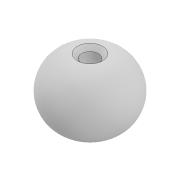
# Autodesk Inventor part: seventh
Saved by Autodesk Inventor 2020 (Build 240168000, 168)
## iProperties
Created: 2021-12-10
Part Number: seventh
Material: Generic
Document SubType Name: Modeling
Designer: NIKHIL VINOD
Density: 1 g/cm^3
Appearance: Default
Author: NIKHIL VINOD
Autodesk Inventor part; units mm, degrees
ref_plane "YZ Plane" through (0, 0, 0) normal (1, 0, 0) x (0, 1, 0)
ref_plane "XZ Plane" through (0, 0, 0) normal (0, 1, 0) x (-1, 0, 0)
ref_plane "XY Plane" through (0, 0, 0) normal (0, 0, 1) x (1, 0, 0)
sketch "Sketch1" plane through (0, 0, 0) normal (0, 0, 1) x (1, 0, 0)
  line L0 (-2, 4.1282) -> (-2, -9.8718)
  line L1 (0, 8.5037) -> (0, -11.0762)
  line L2 (-2, -9.8718) -> (-4, -9.8718)
  line L3 (-3, 5.1282) -> (-2, 4.1282)
  arc A0 (-3, 5.1282) -> (-4, -9.8718) centre (-1.7735, -2.4869) ccw
  point P0 (0, 0)
  dimension "d4" = 2
  dimension "d5" = 0
  dimension "d6" = 2
  constraints: 8 end point, 2 point on circle, 1 centre point, 1 horizontal, 1 point on line, 1 vertical
  measures "d4" distance between parallel lines of L1 L0
  measures "d5" distance from line of point (0, 0) L1
  measures "d6" distance of L0.end L2.end
revolve "Revolution1" add sketch "Sketch1" angle 360 about axis through (0, 8.5037, 0) along (0, -1, 0)
body "Solid1"
